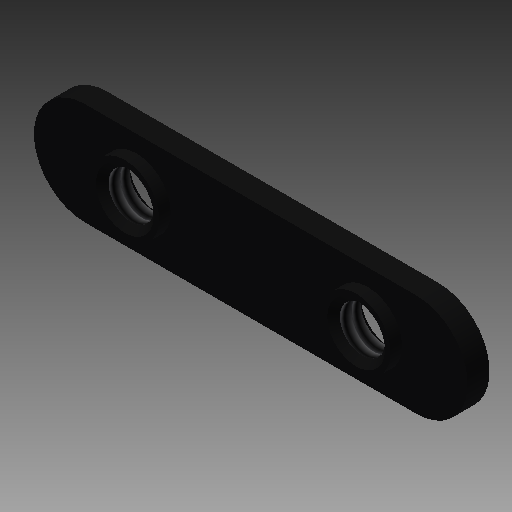
# Autodesk Inventor part: 3280
Saved by Autodesk Inventor 2017 (Build 210142000, 142)
## iProperties
Category: PARTsolutions
Company: 8020
Created: 2017-08-19
Part Number: 3280
Catalog Web Link: www.cadenas.de
Description: 3281, 3280, 3800, 3279, 3879-Double Slide-In Economy T-Nuts
Vendor: 8020
Document SubType Name: Modeling
Designer: psAdmin
Manufacturer: 8020
Mass: 1.18173 g
Surface Area: 13.5311 cm^2
Volume: 1.18173 cm^3
Density: 1 g/cm^3
Material: Generic
Appearance: PSOLRGB-0-0-0
PSOL_IDENT_0: {$CADENAS_DATA\23d-libs\8020\inch\fastening_options\3281.prj},163 {VTYP=3D},{NB=3280},{LINA=3280},{N
PSOL_IDENT_1: N=3281, 3280, 3800, 3279, 3879},{DATE=22.08.2012},{GEOMDATE=09.07.2012 12:28:00},{VERSION=},{LINEID=
PSOL_IDENT_2: 20},{LINESUBID=-1},{WBVAR=}  {NB=3280},{LINA=3280},{KT=DUMMY},{PN=3280},{FIN=Black Zinc},{A=1.875},{
PSOL_IDENT_3: B=0.443},{B1=0.4430},{C=1.000},{D=0.443},{E=1/4-20},{E1=0.2500},{F=0.095},{W=.012},{TT=UNC},{DIA=0.2
PSOL_IDENT_4: 97},{X=0.050},{COL=0.00,0.00,0.00,0.00}
NN: 3281, 3280, 3800, 3279, 3879
NT: Double Slide-In Economy T-Nuts
NB: 3280
NBSYN: $PN.
LINA: 3280
PN: 3280
FIN: Black Zinc
A: 1.875
B: 0.443
C: 1.000
D: 0.443
E: 1/4-20
F: 0.095
W: .012
SUPPLIER: 8020
ARTICLENO: 3280
BOMINFO: 3280
CREATOR: CADENAS GmbH
Title: 3280
Author: Cadenas PARTsolutions
Comments: Double Slide-In Economy T-Nuts
Autodesk Inventor part; units mm, degrees
sketch "Sketch_1" plane through (0, 0, 0) normal (0, 0, 1) x (1, 0, 0)
  arc A0 (-5.6261, 5.6261) -> (-5.6261, -5.6261) centre (-5.6261, 0) ccw
  line L0 (-5.6261, -5.6261) -> (30.7467, -5.6261)
  arc A1 (30.7467, -5.6261) -> (30.7467, 5.6261) centre (30.7467, 0) ccw
  line L1 (30.7467, 5.6261) -> (-5.6261, 5.6261)
  constraints: 4 end point, 4 point on circle, 2 centre point
extrude "Extrusion1" add sketch "Sketch_1" along normal mid plane 2.413
sketch "Sketch_2" plane through (0, 0, 0) normal (0, 1, 0) x (-1, 0, 0)
  line L0 (0, 2.4765) -> (0, -1.2065)
  line L1 (0, -1.2065) -> (-3.7719, -1.2065)
  line L2 (-3.7719, -1.2065) -> (-3.7719, 2.4765)
  line L3 (-3.7719, 2.4765) -> (0, 2.4765)
  line L4 (0, 2.4765) -> (0, -1.2065)
  constraints: 10 end point
revolve "Revolution1" add sketch "Sketch_2" angle 360 about axis through (0, 0, 2.4765) along (0, 0, 1)
sketch "Sketch_3" plane through (0, 0, 0) normal (0, 1, 0) x (-1, 0, 0)
  line L0 (-25.4, 2.4765) -> (-25.4, -1.2065)
  line L1 (-25.4, -1.2065) -> (-29.1719, -1.2065)
  line L2 (-29.1719, -1.2065) -> (-29.1719, 2.4765)
  line L3 (-29.1719, 2.4765) -> (-25.4, 2.4765)
  line L4 (-25.4, 2.4765) -> (-25.4, -1.2065)
  constraints: 10 end point
revolve "Revolution2" add sketch "Sketch_3" angle 360 about axis through (25.4, 0, 2.4765) along (0, 0, 1)
sketch "Sketch_4" plane through (0, 0, 0) normal (0, 1, 0) x (-1, 0, 0)
  line L0 (0, 2.4765) -> (0, -1.2065)
  line L1 (0, -1.2065) -> (-3.175, -1.2065)
  line L2 (-3.175, -1.2065) -> (-2.4879, -0.5194)
  line L3 (-2.4879, -0.5194) -> (-2.4879, 1.7894)
  line L4 (-2.4879, 1.7894) -> (-3.175, 2.4765)
  line L5 (-3.175, 2.4765) -> (0, 2.4765)
  line L6 (0, 2.4765) -> (0, -1.2065)
  constraints: 14 end point
revolve "Revolution3" cut sketch "Sketch_4" angle 360 about axis through (0, 0, 2.4765) along (0, 0, 1)
thread "Thread1" size "1/4-20 UNC" class "2B" standard "ANSI Unified Screw Threads" full length
sketch "Sketch_5" plane through (0, 0, 0) normal (0, 1, 0) x (-1, 0, 0)
  line L0 (-25.4, 2.4765) -> (-25.4, -1.2065)
  line L1 (-25.4, -1.2065) -> (-28.575, -1.2065)
  line L2 (-28.575, -1.2065) -> (-27.8879, -0.5194)
  line L3 (-27.8879, -0.5194) -> (-27.8879, 1.7894)
  line L4 (-27.8879, 1.7894) -> (-28.575, 2.4765)
  line L5 (-28.575, 2.4765) -> (-25.4, 2.4765)
  line L6 (-25.4, 2.4765) -> (-25.4, -1.2065)
  constraints: 14 end point
revolve "Revolution4" cut sketch "Sketch_5" angle 360 about axis through (25.4, 0, 2.4765) along (0, 0, 1)
thread "Thread2" size "1/4-20 UNC" class "2B" standard "ANSI Unified Screw Threads" full length
ref_plane "tnut_XY" through (0, 0, -1.2065) normal (0, 0, 1) x (1, 0, 0)
ref_plane "tnut_YZ" through (0, 0, -1.2065) normal (1, 0, 0) x (0, 1, 0)
ref_plane "tnut_ZX" through (0, 0, -1.2065) normal (0, 1, 0) x (0, 0, 1)
ref_plane "tnut1_XY" through (25.4, 0, -1.2065) normal (0, 0, 1) x (1, 0, 0)
ref_plane "tnut1_YZ" through (25.4, 0, -1.2065) normal (1, 0, 0) x (0, 1, 0)
ref_plane "tnut1_ZX" through (25.4, 0, -1.2065) normal (0, 1, 0) x (0, 0, 1)
body "Solid1"
